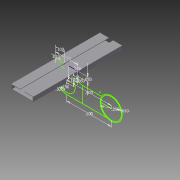
# Autodesk Inventor part: TreadPart1
Saved by Autodesk Inventor 2015 (Build 190159000, 159)
## iProperties
Created: 2015-09-25
Part Number: TreadPart1
Material: Generic
Document SubType Name: Modeling
Designer: mabehnke
Density: 1 g/cm^3
Appearance: Default
Author: mabehnke
Autodesk Inventor part; units mm, degrees
ref_plane "YZ Plane" through (0, 0, 0) normal (1, 0, 0) x (0, 1, 0)
ref_plane "XZ Plane" through (0, 0, 0) normal (0, 1, 0) x (-1, 0, 0)
ref_plane "XY Plane" through (0, 0, 0) normal (0, 0, 1) x (1, 0, 0)
sketch "Sketch1" plane through (0, 0, 0) normal (0, 0, 1) x (1, 0, 0)
  point P0 (0, 0)
sketch "Sketch2" plane through (0, 0, 0) normal (0, 0, 1) x (1, 0, 0)
  line L0 (0, 0) -> (6.35, 0)
  line L1 (6.35, 0) -> (6.35, 1.27)
  line L2 (0, 0) -> (0, 1.27)
  line L3 (0, 1.27) -> (2.54, 1.27)
  line L4 (6.35, 1.27) -> (3.81, 1.27)
  line L5 (2.54, 1.27) -> (2.54, 1.1357)
  line L6 (2.54, 1.1357) -> (0.254, 1.1357)
  line L7 (0.254, 1.1357) -> (0.254, 0.1108)
  line L8 (0.254, 0.1108) -> (6.096, 0.1108)
  line L9 (6.096, 0.1108) -> (6.096, 1.1357)
  line L10 (6.096, 1.1357) -> (3.81, 1.1357)
  line L11 (3.81, 1.1357) -> (3.81, 1.27)
  line L12 (0.254, -3.175) -> (0.254, 0)
  circle A0 centre (15.875, -3.175) radius 3.175
  circle A1 centre (15.875, -3.175) radius 2.921
  line L13 (3.1985, -6.0959) -> (15.8985, -6.0959)
  arc A2 (0.254, -3.175) -> (0.2538, -3.175) centre (0.2539, -5.715) ccw
  line L14 (0.254, -4.0044) -> (0.254, -4.0014)
  line L15 (0.254, -3.175) -> (0.254, -3.175)
  circle A3 centre (3.175, -3.175) radius 2.413
  arc A4 (0.254, -3.175) -> (3.1985, -6.0959) centre (3.175, -3.175) ccw
  line L16 (6.096, 0) -> (6.096, -0.1394)
  line L17 (7.5457, -1.5893) -> (12.7523, -1.5893)
  arc A5 (12.7523, -1.5893) -> (13.4637, -1.1095) centre (12.7523, -0.822) ccw
  arc A6 (6.096, 0) -> (7.6855, -1.5893) centre (7.6156, -0.0697) ccw
  line L18 (7.6855, -1.5893) -> (7.6855, -6.0959)
  line L19 (3.175, -3.175) -> (3.81, -3.175)
  line L20 (12.7, -3.175) -> (15.875, -3.175)
  point P0 (3.1515, -6.0959)
  dimension "d1" = 6.35
  dimension "d2" = 1.27
  dimension "d6" = 2.54
  dimension "d7" = 2.54
  dimension "d11" = 12.7
  dimension "d14" = 12.7
  dimension "d16" = 0.254
  dimension "d17" = 0.254
  dimension "d18" = 6.35
  dimension "d21" = 0.254
  dimension "d22" = 4.826
  dimension "d23" = 0.508
  dimension "d24" = 3.175
  dimension "d25" = 1.5212
  constraints: 42 end point, 13 point on circle, 10 perpendicular, 8 point on line, 6 centre point, 5 horizontal, 5 vertical, 3 coincident, 3 tangent, 1 horizontal alignment, 5 other
  measures "d1" distance of L0.start L0.end
  measures "d2" distance of L0.end L1.end
  measures "d6" distance of L2.end L3.end
  measures "d7" distance of L1.end L4.end
  measures "d11" distance of L19.start L20.end
  measures "d14" distance of L13.start L13.end
  measures "d16" distance between parallel lines of L1 L9
  measures "d17" distance between parallel lines of L2 L7
  measures "d18" diameter of A0
  measures "d22" diameter of A3
  measures "d23" radial gap between concentric circles of A4 A3
  measures "d24" distance from line of L0 A3.centre
  measures "d25" radius of A6
extrude "Extrusion1" add sketch "Sketch2" along normal blind 12.7 contours L2 L3 L5 L6 L7 L8 L9 L10 L11 L4 L1 L0
extrude "Extrusion2" add sketch "Sketch2" against normal blind 12.7 contours L2 L3 L5 L6 L7 L8 L9 L10 L11 L4 L1 L0
body "Solid1"
